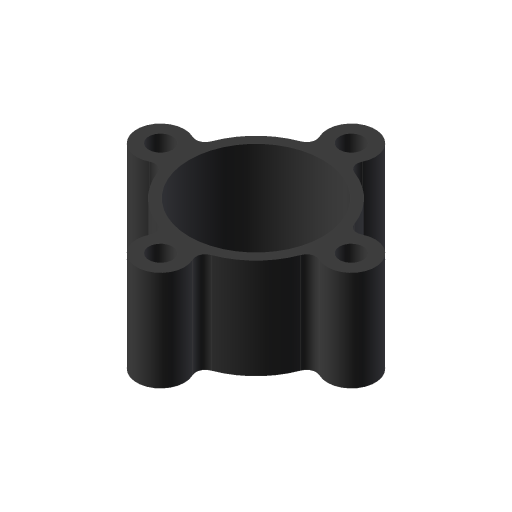
# Autodesk Inventor part: PDMS_insert
Saved by Autodesk Inventor 2023 (Build 270158000, 158)
## iProperties
Created: 2026-03-05
Part Number: PDMS_insert
Material: Generic
Document SubType Name: Modeling
Designer: ferrerx
Density: 1 g/cm^3
Appearance: Default
Author: ferrerx
Autodesk Inventor part; units mm, degrees
ref_plane "YZ Plane" through (0, 0, 0) normal (1, 0, 0) x (0, 1, 0)
ref_plane "XZ Plane" through (0, 0, 0) normal (0, 1, 0) x (-1, 0, 0)
ref_plane "XY Plane" through (0, 0, 0) normal (0, 0, 1) x (1, 0, 0)
sketch "Sketch1" plane through (0, 0, 0) normal (0, 1, 0) x (-1, 0, 0)
  circle A0 centre (0, 0) radius 7
  circle A1 centre (0, 0) radius 8
  dimension "d0" = 14
  dimension "d1" = 1
  constraints: 2 centre point, 2 coincident
  measures "d0" diameter of A0
  measures "d1" radial gap between concentric circles of A0 A1
extrude "Extrusion1" add sketch "Sketch1" along normal blind 10.5
sketch "Sketch2" plane through (0, 0, 0) normal (0, -1, 0) x (1, 0, 0)
  circle A0 centre (0, 0) radius 8
  constraints: 1 centre point, 1 coincident
extrude "Extrusion2" add sketch "Sketch2" against normal blind 0.5
sketch "Sketch4" plane through (0, 10.5, 0) normal (0, 1, 0) x (1, 0, 0)
  circle A0 centre (-10, 0) radius 1.25
  circle A1 centre (-10, 0) radius 2.5
  point P0 (0, 0)
  dimension "d6" = 5
  dimension "d7" = 2.5
  dimension "d8" = 10
  constraints: 2 centre point, 1 coincident
  measures "d6" diameter of A1
  measures "d7" diameter of A0
  measures "d8" distance of point (0, 0) A1.centre
extrude "Extrusion3" add sketch "Sketch4" against normal up to surface (10.5 mm away)
pattern_circular "Circular Pattern1" count 4 over 360 about axis through (0, 0, 0) along (0, 1, 0) of "Extrusion3"
fillet "Fillet1" radius 1 8 edges at (7.8875, 5.25, -1.3369) (7.8875, 5.25, 1.3369) (1.3369, 5.25, 7.8875) (-1.3369, 5.25, 7.8875) (-7.8875, 5.25, 1.3369) (-7.8875, 5.25, -1.3369) (-1.3369, 5.25, -7.8875) (1.3369, 5.25, -7.8875)
body "Solid1"
